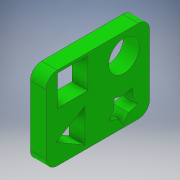
# Autodesk Inventor part: Passenger base
Saved by Autodesk Inventor 2017 (Build 210142000, 142)
## iProperties
Created: 2016-11-14
Part Number: Passenger base
Material: Generic
Document SubType Name: Modeling
Designer: rbibb
Density: 1 g/cm^3
Appearance: Default
Author: rbibb
Autodesk Inventor part; units mm, degrees
ref_plane "YZ Plane" through (0, 0, 0) normal (1, 0, 0) x (0, 1, 0)
ref_plane "XZ Plane" through (0, 0, 0) normal (0, 1, 0) x (-1, 0, 0)
ref_plane "XY Plane" through (0, 0, 0) normal (0, 0, 1) x (1, 0, 0)
sketch "Sketch1" plane through (0, 0, 0) normal (1, 0, 0) x (0, 1, 0)
  line L0 (4.3954, 24.8951) -> (-24.8146, 24.8951)
  line L1 (-30.2756, 19.4341) -> (-30.2756, -19.8089)
  line L2 (-24.8146, -25.2699) -> (4.3954, -25.2699)
  line L3 (9.8564, -19.8089) -> (9.8564, 19.4341)
  arc A0 (4.3954, -25.2699) -> (9.8564, -19.8089) centre (4.3954, -19.8089) ccw
  arc A1 (9.8564, 19.4341) -> (4.3954, 24.8951) centre (4.3954, 19.4341) ccw
  arc A2 (-30.2756, -19.8089) -> (-24.8146, -25.2699) centre (-24.8146, -19.8089) ccw
  arc A3 (-24.8146, 24.8951) -> (-30.2756, 19.4341) centre (-24.8146, 19.4341) ccw
  point P0 (0, 0)
  point P1 (-30.2756, -25.2699)
  point P2 (-30.2756, 24.8951)
  point P3 (9.8564, -25.2699)
  dimension "d0" = 40.132
  dimension "d1" = 50.165
  dimension "d2" = 5.461
  dimension "d3" = 5.461
  constraints: 8 end point, 8 point on circle, 8 tangent, 6 point on line, 4 centre point, 2 equal radius, 2 parallel, 1 horizontal, 1 perpendicular
  measures "d0" distance of point (9.856, -25.27) point (-30.276, -25.27)
  measures "d1" distance of point (-30.276, -25.27) point (-30.276, 24.895)
  measures "d2" radius of A0
  measures "d3" radius of A1
extrude "Extrusion1" add sketch "Sketch1" along normal blind 7.62
sketch "Sketch2" plane through (0, 0, 0) normal (-1, 0, 0) x (0, 0, 1)
  line L0 (-25.2699, -24.8146) -> (-25.2699, 4.3954) projected
  line L1 (-25.2699, 4.3954) -> (-20.1899, 4.3954)
  line L2 (-20.1899, 4.3954) -> (-20.1899, 9.8564)
  line L3 (19.4341, 9.8564) -> (-19.8089, 9.8564) projected
  line L4 (-20.1899, 7.1259) -> (-5.4579, 7.1259)
  line L5 (-5.4579, 7.1259) -> (-5.4579, -7.6061)
  line L6 (-5.4579, -7.6061) -> (-20.1899, -7.6061)
  line L7 (-20.1899, -7.6061) -> (-20.1899, 7.1259)
  circle A0 centre (-12.8239, -0.2401) radius 7.366
  point P0 (0, 0)
  dimension "d6" = 5.08
  dimension "d7" = 14.732
  dimension "d8" = 14.732
  dimension "d9" = 14.732
  constraints: 12 end point, 3 tangent, 2 horizontal, 2 perpendicular, 2 point on line, 1 centre point, 1 collinear, 1 midpoint
  measures "d6" distance of L0.end L1.end
  measures "d7" distance of L4.start L4.end
  measures "d8" distance of L4.end L5.end
  measures "d9" distance of L5.end L6.end
extrude "Extrusion2" cut sketch "Sketch2" against normal up to next contours A0
sketch "Sketch3" plane through (0, 0, 0) normal (-1, 0, 0) x (0, 0, 1)
  point P0 (0, 0)
sketch "Sketch4" plane through (0, 0, 0) normal (-1, 0, 0) x (0, 0, 1)
  arc A0 (24.8951, 4.3954) -> (19.4341, 9.8564) centre (19.8306, 4.7919) ccw
  line L0 (19.4341, 9.8564) -> (19.4341, 8.5864)
  line L1 (19.4341, 8.5864) -> (4.7021, 8.5864)
  line L2 (4.7021, 8.5864) -> (4.7021, -6.1456)
  line L3 (4.7021, -6.1456) -> (19.4341, -6.1456)
  line L4 (19.4341, -6.1456) -> (19.4341, 8.5864)
  point P0 (0, 0)
  dimension "d13" = 1.27
  dimension "d14" = 14.732
  dimension "d15" = 14.732
  constraints: 10 end point, 2 parallel, 2 point on circle, 1 centre point, 1 horizontal, 1 perpendicular, 1 vertical
  measures "d13" distance of L0.start L0.end
  measures "d14" distance of L3.end L2.end
  measures "d15" distance of L2.end L1.end
extrude "Extrusion3" cut sketch "Sketch4" against normal up to next
sketch "Sketch5" plane through (0, 0, 0) normal (-1, 0, 0) x (0, 0, 1)
  line L0 (20.1796, -20.03) -> (6.1455, -28.1326)
  line L1 (6.1455, -28.1326) -> (6.1455, -11.9274)
  line L2 (6.1455, -11.9274) -> (20.1796, -20.03)
  line L3 (4.3902, -29.2503) -> (21.3615, -29.2503)
  point P0 (0, 0)
  point P1 (10.8235, -20.03)
  dimension "d18" = 16.2052
  constraints: 8 end point, 1 horizontal, 1 perpendicular, 7 other
  measures "d18" distance of L1.end L0.start
extrude "Extrusion4" cut sketch "Sketch5" against normal up to next
sketch "Sketch6" plane through (0, 0, 0) normal (-1, 0, 0) x (0, 0, 1)
  line L0 (19.4341, -30.2756) -> (-19.8089, -30.2756) projected
  line L1 (-24.8889, -30.2756) -> (-19.8089, -30.2756)
  line L2 (-19.8089, -30.2756) -> (-19.8089, -29.0056)
  line L3 (-19.8089, -29.0056) -> (-5.0769, -29.0056) construction
  line L4 (-5.0769, -29.0056) -> (-5.0769, -14.2736)
  line L5 (-5.0769, -14.2736) -> (-19.8089, -14.2736) construction
  line L6 (-19.8089, -14.2736) -> (-19.8089, -29.0056) construction
  circle A0 centre (-12.47, -21.7171) radius 7.4436 construction
  line L7 (-8.0948, -15.6951) -> (-5.3908, -24.0173) construction
  line L8 (-5.3908, -24.0173) -> (-12.47, -29.1607) construction
  line L9 (-12.47, -29.1607) -> (-19.5493, -24.0173) construction
  line L10 (-19.5493, -24.0173) -> (-16.8452, -15.6951) construction
  line L11 (-16.8452, -15.6951) -> (-8.0948, -15.6951) construction
  line L12 (-12.47, -21.7171) -> (-5.3908, -24.0173) construction
  line L13 (-12.47, -21.7171) -> (-8.0948, -15.6951) construction
  line L14 (-12.47, -21.7171) -> (-16.8452, -15.6951) construction
  line L15 (-12.47, -21.7171) -> (-19.5493, -24.0173) construction
  line L16 (-16.8452, -15.6951) -> (-11.847, -15.6951) construction
  line L17 (-12.47, -29.1607) -> (-7.7202, -29.1607) construction
  line L18 (-12.47, -21.7171) -> (-12.47, -29.1607) construction
  line L19 (-12.47, -21.7171) -> (-6.7428, -19.8562) construction
  line L20 (-8.0948, -15.6951) -> (-7.9391, -20.2449)
  line L21 (-7.9391, -20.2449) -> (-5.3908, -24.0173)
  line L22 (-12.47, -21.7171) -> (-8.9304, -26.589) construction
  line L23 (-5.3908, -24.0173) -> (-9.9432, -25.195)
  line L24 (-12.47, -29.1607) -> (-9.9432, -25.195)
  line L25 (-12.47, -21.7171) -> (-16.0096, -26.589) construction
  line L26 (-12.47, -21.7171) -> (-18.666, -19.7714) construction
  line L27 (-12.47, -21.7171) -> (-12.4334, -15.6951) construction
  line L28 (-19.5493, -24.0173) -> (-16.8734, -20.3343)
  line L29 (-16.8452, -15.6951) -> (-16.8734, -20.3343)
  line L30 (-16.8452, -15.6951) -> (-12.4404, -16.8346)
  line L31 (-12.4404, -16.8346) -> (-8.0948, -15.6951)
  line L32 (-19.5493, -24.0173) -> (-14.9968, -25.195)
  line L33 (-14.9968, -25.195) -> (-12.47, -29.1607)
  point P0 (0, 0)
  point P1 (-12.2672, -15.6951)
  dimension "d21" = 5.08
  dimension "d22" = 1.27
  dimension "d23" = 14.732
  dimension "d24" = 14.732
  dimension "d33" = 4.5524
  dimension "d34" = 4.5524
  constraints: 66 end point, 8 point on line, 5 horizontal, 4 parallel, 3 midpoint, 3 perpendicular, 2 equal length, 1 coincident, 1 collinear, 1 vertical, 14 other
  measures "d21" distance of L1.start L0.end
  measures "d22" distance of L0.end L2.end
  measures "d23" distance of L5.end L4.end
  measures "d24" distance of L4.end L3.end
  measures "d33" distance of L7.start L20.end
  measures "d34" horizontal distance of L21.end L23.end
sketch "Sketch7" plane through (0, 0, 0) normal (-1, 0, 0) x (0, 0, 1)
  point P0 (0, 0)
sketch "Sketch8" plane through (0, 0, 0) normal (-1, 0, 0) x (0, 0, 1)
  point P0 (0, 0)
sketch "Sketch9" plane through (0, 0, 0) normal (-1, 0, 0) x (0, 0, 1)
  point P0 (0, 0)
extrude "Extrusion5" cut sketch "Sketch6" against normal up to next
body "Solid1"
